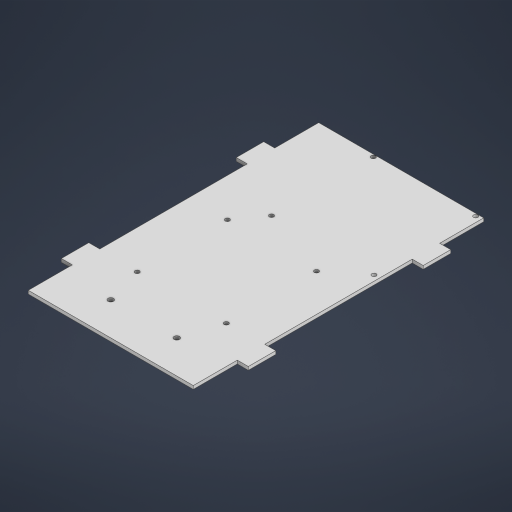
# Autodesk Inventor part: bottom_part
Saved by Autodesk Inventor 2023 (Build 270158000, 158)
## iProperties
Created: 2022-11-27
Part Number: bottom_part
Material: Generic
Document SubType Name: Modeling
Designer: washington
Density: 1 g/cm^3
Appearance: Default
Author: washington
Autodesk Inventor part; units mm, degrees
ref_plane "YZ Plane" through (0, 0, 0) normal (1, 0, 0) x (0, 1, 0)
ref_plane "XZ Plane" through (0, 0, 0) normal (0, 1, 0) x (-1, 0, 0)
ref_plane "XY Plane" through (0, 0, 0) normal (0, 0, 1) x (1, 0, 0)
sketch "Sketch1" plane through (0, 0, 0) normal (0, 1, 0) x (-1, 0, 0)
  line L0 (75, 132) -> (-75, 132)
  line L1 (-75, -132) -> (75, -132)
  line L2 (75, 132) -> (-75, -132) construction
  line L3 (-75, 132) -> (75, -132) construction
  line L4 (75, 92) -> (85, 92)
  line L5 (85, 92) -> (85, 67)
  line L6 (85, 67) -> (75, 67)
  line L7 (75, 92) -> (75, 132)
  line L8 (0, 0) -> (94, 0)
  line L9 (75, -92) -> (85, -92)
  line L10 (85, -92) -> (85, -67)
  line L11 (85, -67) -> (75, -67)
  line L12 (75, -132) -> (75, -92)
  line L13 (75, -67) -> (75, 67)
  line L14 (-75, 92) -> (-85, 92)
  line L15 (-85, 92) -> (-85, 67)
  line L16 (-85, 67) -> (-75, 67)
  line L17 (-75, 132) -> (-75, 92)
  line L18 (-75, -92) -> (-85, -92)
  line L19 (-85, -92) -> (-85, -67)
  line L20 (-85, -67) -> (-75, -67)
  line L21 (-75, 67) -> (-75, -67)
  line L22 (-75, -92) -> (-75, -132)
  circle A0 centre (30, 102) radius 2.5
  circle A1 centre (-30, 102) radius 2.5
  dimension "d0" = 264
  dimension "d1" = 150
  dimension "d4" = 10
  dimension "d5" = 25
  dimension "d6" = 40
  dimension "d7" = 10
  dimension "d8" = 9
  dimension "d9" = 10
  dimension "d10" = 25
  dimension "d11" = 40
  dimension "d12" = 160
  dimension "d17" = 5
  dimension "d18" = 5
  dimension "d19" = 30
  dimension "d20" = 30
  dimension "d21" = 45
  dimension "d22" = 45
  constraints: 46 end point, 11 perpendicular, 10 parallel, 8 symmetric about line, 4 horizontal, 2 centre point, 2 midpoint
  measures "d0" distance of L0.end L1.start
  measures "d1" distance of L1.start L1.end
  measures "d4" distance of L4.start L4.end
  measures "d5" distance of L4.end L5.end
  measures "d6" distance of L0.start L4.start
  measures "d7" distance between parallel lines of L13 L5
  measures "d8" distance from line of L8.end L5
  measures "d9" distance of L14.start L14.end
  measures "d10" distance of L14.end L15.end
  measures "d11" vertical distance of L0.end L14.end
  measures "d12" distance between parallel lines of L21 L5
  measures "d17" diameter of A1
  measures "d18" diameter of A0
  measures "d19" vertical distance of L0.end A1.centre
  measures "d20" vertical distance of L0.start A0.centre
  measures "d21" horizontal distance of L0.end A1.centre
  measures "d22" distance from line of A0.centre L13
extrude "Extrusion1" add sketch "Sketch1" along normal blind 3
sketch "Sketch2" plane through (0, 3, 0) normal (0, 1, 0) x (1, 0, 0)
  line L0 (-86, -72) -> (86, -72)
  line L1 (-75, -132) -> (75, -132) projected
  line L2 (45, -72) -> (45, 18)
  line L3 (75, -67) -> (75, 67) projected
  line L4 (45, 18) -> (-44, 18)
  line L5 (-44, 18) -> (-44, -72)
  line L6 (-75, 67) -> (-75, -67) projected
  circle A0 centre (41, -68) radius 2
  circle A1 centre (41, 14) radius 2
  circle A2 centre (-40, 14) radius 2
  circle A3 centre (-40, -68) radius 2
  circle A4 centre (70, 129.734) radius 2
  line L7 (75, 132) -> (-75, 132) projected
  circle A5 centre (70, 37.266) radius 2
  circle A6 centre (-23.148, 129.734) radius 2
  circle A7 centre (-23.148, 37.266) radius 2
  point P0 (0, 0)
  dimension "d15" = 60
  dimension "d16" = 30
  dimension "d23" = 90
  dimension "d25" = 4
  dimension "d26" = 4
  dimension "d27" = 4
  dimension "d28" = 4
  dimension "d29" = 4
  dimension "d30" = 4
  dimension "d31" = 4
  dimension "d32" = 4
  dimension "d33" = 4
  dimension "d34" = 4
  dimension "d35" = 4
  dimension "d36" = 4
  dimension "d39" = 89
  dimension "d40" = 4
  dimension "d41" = 5
  dimension "d42" = 2.266
  dimension "d43" = 4
  dimension "d44" = 5
  dimension "d45" = 92.468
  dimension "d46" = 4
  dimension "d47" = 4
  dimension "d48" = 93.148
  dimension "d49" = 93.148
  dimension "d50" = 2.266
  dimension "d51" = 0
  constraints: 8 centre point, 8 end point, 2 horizontal, 2 point on line, 1 perpendicular, 1 vertical
  measures "d15" distance between parallel lines of L0 L1
  measures "d16" distance between parallel lines of L2 L3
  measures "d23" distance of L2.start L2.end
  measures "d25" distance from line of A0.centre L2
  measures "d26" distance from line of L0 A0.centre
  measures "d27" diameter of A0
  measures "d28" distance from line of A1.centre L2
  measures "d29" distance from line of L4 A1.centre
  measures "d30" diameter of A1
  measures "d31" distance from line of L4 A2.centre
  measures "d32" distance from line of L5 A2.centre
  measures "d33" diameter of A2
  measures "d34" distance from line of L0 A3.centre
  measures "d35" distance from line of L5 A3.centre
  measures "d36" diameter of A3
  measures "d39" distance between parallel lines of L5 L2
  measures "d40" diameter of A4
  measures "d41" distance from line of L3 A4.centre
  measures "d42" distance from line of L7 A4.centre
  measures "d43" diameter of A5
  measures "d44" distance from line of A5.centre L3
  measures "d45" distance of A4.centre A5.centre
  measures "d46" diameter of A6
  measures "d47" diameter of A7
  measures "d48" distance of A6.centre A4.centre
  measures "d49" distance of A7.centre A5.centre
  measures "d50" distance from line of L7 A6.centre
  measures "d51" vertical distance of A7.centre A5.centre
extrude "Extrusion2" cut sketch "Sketch2" against normal blind 3 contours A0 | A1 | A2 | A3 | A4 | A5 | A6 | A7
body "Solid1"
